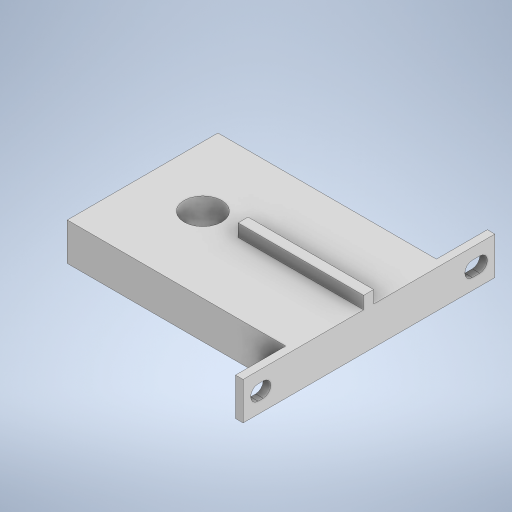
# Autodesk Inventor part: Стенка энкодера штурвала
Saved by Autodesk Inventor 2023 (Build 270158000, 158)
## iProperties
Created: 2022-05-17
Part Number: Стенка энкодера штурвала
Material: Типовые
Document SubType Name: Modeling
Designer: avkap
Density: 1 g/cm^3
Appearance: По умолчанию
Author: avkap
Autodesk Inventor part; units mm, degrees
ref_plane "YZ Plane" through (0, 0, 0) normal (1, 0, 0) x (0, 1, 0)
sketch "Эскиз1" plane through (0, 0, 0) normal (0, 1, 0) x (-1, 0, 0)
  line L0 (0, 0) -> (90, 0)
  line L1 (90, 0) -> (90, -60)
  line L2 (90, -60) -> (0, -60)
  line L3 (0, -60) -> (0, 0)
  line L4 (0, -60) -> (66, -60)
  line L5 (0, -30) -> (66, -30)
  circle A0 centre (66, -30) radius 7.5
  dimension "d0" = 90
  dimension "d1" = 60
  dimension "d67" = 66
  dimension "d68" = 15
  constraints: 12 end point, 2 horizontal, 2 parallel, 1 centre point, 1 coincident, 1 midpoint, 1 perpendicular, 1 point on line
  measures "d0" distance of L1.end L2.end
  measures "d1" distance of L0.end L1.end
  measures "d67" distance of L5.start L5.end
  measures "d68" diameter of A0
extrude "Выдавливание1" add sketch "Эскиз1" along normal blind 15
ref_plane "РабПлоскость3" through (0, 15, 0) normal (0, 1, 0) x (1, 0, 0)
sketch "Эскиз3" plane through (0, 15, 0) normal (0, 1, 0) x (1, 0, 0)
  line L0 (0, 0) -> (0, 60) projected
  line L1 (0, 30) -> (0, 28)
  line L2 (0, 28) -> (-50, 28)
  line L3 (-50, 28) -> (-50, 32)
  line L4 (-50, 32) -> (0, 32)
  line L5 (0, 32) -> (0, 28)
  point P0 (0, 32)
  dimension "d13" = 2
  dimension "d14" = 50
  dimension "d15" = 4
  constraints: 10 end point, 2 perpendicular, 2 point on line, 1 midpoint
  measures "d13" distance of L1.start L1.end
  measures "d14" distance of L1.end L2.end
  measures "d15" distance of L2.end L3.end
extrude "Выдавливание3" add sketch "Эскиз3" along normal blind 5
ref_plane "РабПлоскость1" through (0, 15, 0) normal (0, 1, 0) x (1, 0, 0)
sketch "Эскиз6" plane through (0, 15, 0) normal (0, 1, 0) x (1, 0, 0)
  circle A0 centre (-66, 30) radius 7.5 projected
  line L0 (-66, 30) -> (-66, -120)
  line L1 (-150, -120) -> (0, -120) projected
  line L2 (-66, -120) -> (-66, -100)
  circle A1 centre (-66, -100) radius 10
  circle A2 centre (-66, -100) radius 20
  circle A3 centre (-66, 30) radius 40
  line L3 (-85.7619, -103.0769) -> (-105.5238, 23.8462)
  line L4 (-46.2381, -103.0769) -> (-26.4762, 23.8462)
  line L5 (-66, -100) -> (-66, -40)
  line L6 (-66, -40) -> (-91, -40)
  line L7 (-66, -40) -> (-41, -40)
  circle A4 centre (-91, -40) radius 2.5
  circle A5 centre (-41, -40) radius 2.5
  point P0 (0, 0)
  dimension "d45" = 20
  dimension "d46" = 20
  dimension "d47" = 40
  dimension "d48" = 80
  dimension "d49" = 60
  dimension "d50" = 25
  dimension "d52" = 25
  dimension "d53" = 5
  dimension "d54" = 5
  constraints: 14 end point, 5 centre point, 5 coincident, 4 point on circle, 4 tangent, 3 point on line, 1 perpendicular, 1 vertical
  measures "d45" distance of L0.end L2.end
  measures "d46" diameter of A1
  measures "d47" diameter of A2
  measures "d48" diameter of A3
  measures "d49" distance of L5.start L5.end
  measures "d50" distance of L5.end L6.end
  measures "d52" distance of L5.end L7.end
  measures "d53" diameter of A4
  measures "d54" diameter of A5
sketch "Эскиз7" plane through (0, 0, 0) normal (1, 0, 0) x (0, 0, -1)
  line L0 (80.2787, 0) -> (80.2787, 15)
  line L1 (60, 15) -> (0, 15) projected
  line L2 (80.2787, 15) -> (60.2787, 15)
  line L3 (60.2787, 15) -> (0, 15)
  line L4 (0, 0) -> (0, 15) projected
  line L5 (0, 15) -> (-20, 15)
  line L6 (-20, 15) -> (-20, 0)
  line L7 (-20, 0) -> (0, 0)
  line L8 (-20, 7.5) -> (-14, 7.5)
  line L9 (80.2787, 7.5) -> (74.2787, 7.5)
  arc A0 (74.2787, 4.5) -> (74.2787, 10.5) centre (74.2787, 7.5) ccw
  arc A1 (-14, 10.5) -> (-14, 4.5) centre (-14, 7.5) ccw
  line L10 (60, 0) -> (0, 0) projected
  line L11 (60, 0) -> (0, 0)
  line L12 (60, 0) -> (60, 15) projected
  line L13 (60, 0) -> (60, 15)
  line L14 (60, 0) -> (80.2787, 0)
  line L15 (74.2787, 4.5) -> (71.2787, 4.5)
  line L16 (71.2787, 10.5) -> (74.2787, 10.5)
  arc A2 (71.2787, 10.5) -> (71.2787, 4.5) centre (71.2787, 7.5) ccw
  line L17 (-14, 7.5) -> (-12, 7.5)
  arc A3 (-12, 4.5) -> (-12, 10.5) centre (-12, 7.5) ccw
  line L18 (-14, 7.5) -> (-14, 10.5)
  line L19 (-14, 10.5) -> (-12, 10.5)
  line L20 (-14, 4.5) -> (-12, 4.5)
  point P0 (-17, 7.5)
  dimension "d59" = 20
  dimension "d60" = 6
  dimension "d61" = 6
  dimension "d62" = 6
  dimension "d63" = 6
  constraints: 34 end point, 8 point on circle, 4 centre point, 4 horizontal, 4 perpendicular, 4 tangent, 3 collinear, 2 coincident, 2 midpoint, 2 point on line, 1 parallel, 1 vertical
  measures "d59" distance of L1.end L5.end
  measures "d60" distance of L8.end L8.start
  measures "d61" distance of L9.start L9.end
  measures "d62" diameter of A0
  measures "d63" diameter of A1
extrude "Выдавливание7" add sketch "Эскиз7" against normal blind 3
